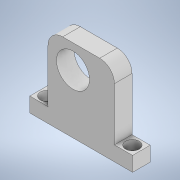
# Autodesk Inventor part: Updated Support_chris
Saved by Autodesk Inventor 2022 (Build 260153000, 153)
## iProperties
Created: 2022-01-29
Part Number: Updated Support_chris
Material: Generic
Document SubType Name: Modeling
Designer: legob
Density: 1 g/cm^3
Appearance: Default
Author: legob
Autodesk Inventor part; units mm, degrees
ref_plane "YZ Plane" through (0, 0, 0) normal (1, 0, 0) x (0, 1, 0)
ref_plane "XZ Plane" through (0, 0, 0) normal (0, 1, 0) x (-1, 0, 0)
ref_plane "XY Plane" through (0, 0, 0) normal (0, 0, 1) x (1, 0, 0)
sketch "Sketch1" plane through (0, 0, 0) normal (0, 0, 1) x (1, 0, 0)
  line L0 (0, 0) -> (88.9, 0)
  line L1 (88.9, 0) -> (88.9, 12.7)
  line L2 (0, 12.7) -> (0, 0)
  line L3 (0, 12.7) -> (0, 0)
  circle A0 centre (37.338, 50.8) radius 14.2875
  line L4 (0, 0) -> (0, 12.7)
  line L5 (0, 0) -> (0, 12.7)
  line L6 (0, 12.7) -> (15.748, 12.7)
  line L7 (13.208, 0) -> (0, 0)
  line L8 (15.748, 12.7) -> (0, 12.7)
  line L9 (15.748, 54.61) -> (15.748, 12.7)
  line L10 (88.9, 0) -> (62.992, 0)
  line L11 (73.152, 12.7) -> (88.9, 12.7)
  line L12 (88.9, 12.7) -> (88.9, 0)
  line L13 (73.152, 12.7) -> (73.152, 54.61)
  line L14 (60.452, 71.222) -> (28.448, 71.222)
  line L15 (15.748, 54.61) -> (15.748, 58.522)
  line L16 (73.152, 58.522) -> (73.152, 54.61)
  arc A1 (28.448, 71.222) -> (15.748, 58.522) centre (28.448, 58.522) ccw
  arc A2 (73.152, 58.522) -> (60.452, 71.222) centre (60.452, 58.522) ccw
  point P0 (65.9232, 76.2)
  point P1 (0, 12.7)
  dimension "d9" = 28.575
  dimension "d10" = 88.9
  dimension "d56" = 12.7
  dimension "d57" = 15.748
  dimension "d79" = 21.59
  dimension "d83" = 15.748
  dimension "d87" = 12.7
  dimension "d111" = 41.91
  dimension "d112" = 41.91
  dimension "d118" = 25.4
  dimension "d119" = 12.7
  constraints: 34 end point, 4 point on circle, 4 tangent, 3 centre point, 3 horizontal, 3 parallel, 3 perpendicular, 1 collinear, 1 point on line, 1 vertical
  measures "d9" diameter of A0
  measures "d10" distance of L0.start L0.end
  measures "d56" distance of L2.start L0.start
  measures "d57" distance of L2.start L6.end
  measures "d79" distance from line of A0.centre L9
  measures "d83" distance of L1.end L11.start
  measures "d87" distance of L0.end L1.end
  measures "d111" distance of L9.start L6.end
  measures "d112" distance of L11.start L13.end
  measures "d118" diameter of A1
  measures "d119" radius of A2
extrude "Extrusion7" add sketch "Sketch1" along normal blind 15.24
sketch "Sketch9" plane through (73.152, 12.7, 0) normal (0, 1, 0) x (1, 0, 0)
  point P0 (-73.152, 0)
  point P1 (8.0463, -7.7031)
hole "Hole4" at (81.1983, 12.7, 7.7031) direction (0, -1, 0) diameter 6.4008 end through all counterbore diameter 11.9062 counterbore depth 7.9502
sketch "Sketch10" plane through (0.0713, 12.7, -0.0767) normal (0, 1, 0) x (1, 0, 0)
  point P0 (-75.692, 0)
  point P1 (7.4278, -7.7745)
hole "Hole5" at (7.4991, 12.7, 7.6977) direction (0, -1, 0) diameter 6.4008 end through all counterbore diameter 11.9062 counterbore depth 7.9502
body "Solid2"
